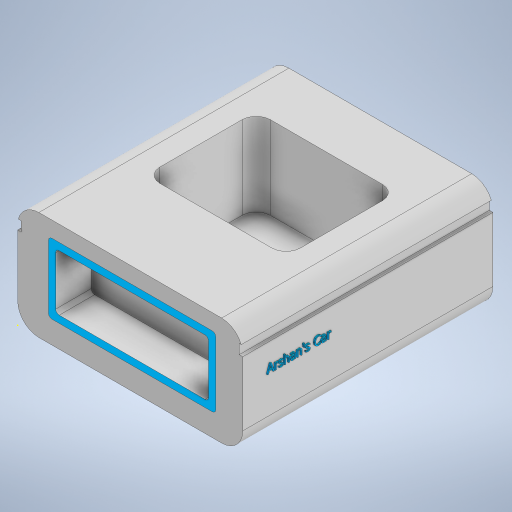
# Autodesk Inventor part: boxthing
Saved by Autodesk Inventor 2023 (Build 270158000, 158)
## iProperties
Created: 2023-08-29
Part Number: boxthing
Material: Generic
Document SubType Name: Modeling
Designer: 1908174
Density: 1 g/cm^3
Appearance: Default
Author: 1908174
Autodesk Inventor part; units mm, degrees
note: some values were not read from the file. Chosen so that the rebuilt part matches the saved one: direction of "Emboss1".
ref_plane "YZ Plane" through (0, 0, 0) normal (1, 0, 0) x (0, 1, 0)
ref_plane "XZ Plane" through (0, 0, 0) normal (0, 1, 0) x (-1, 0, 0)
ref_plane "XY Plane" through (0, 0, 0) normal (0, 0, 1) x (1, 0, 0)
sketch "Sketch2" plane through (0, 0, 0) normal (0, 1, 0) x (-1, 0, 0)
  line L0 (0, -89.780498) -> (-81.1276, -89.780498)
  line L1 (-81.1276, -89.780498) -> (-81.1276, 0.338702)
  line L2 (-81.1276, 0.338702) -> (0, 0.338702)
  line L3 (0, 0.338702) -> (0, -89.780498)
  point P0 (0, 0)
  dimension "d0" = 81.1276
  dimension "d1" = 90.1192
  constraints: 8 end point, 2 parallel, 1 horizontal, 1 perpendicular
  measures "d0" distance of L1.end L2.end
  measures "d1" distance of L0.end L1.end
extrude "Extrusion1" add sketch "Sketch2" along normal blind 39.0144
sketch "Sketch3" plane through (0, 39.0144, 0) normal (0, 1, 0) x (1, 0, 0)
  line L0 (15.2654, 70.349498) -> (65.8368, 70.349498)
  line L1 (65.8368, 70.349498) -> (65.8368, 30.573098)
  line L2 (65.8368, 30.573098) -> (15.2654, 30.573098)
  line L3 (15.2654, 30.573098) -> (15.2654, 70.349498)
  line L4 (0, -0.338702) -> (81.1276, -0.338702)
  line L5 (81.1276, -0.338702) -> (81.1276, 89.780498)
  point P0 (0, 0)
  dimension "d4" = 50.5714
  dimension "d5" = 39.7764
  dimension "d6" = 30.9118
  dimension "d7" = 15.2908
  constraints: 8 end point, 2 parallel, 1 horizontal, 1 perpendicular
  measures "d4" distance of L1.end L2.end
  measures "d5" distance of L0.end L1.end
  measures "d6" distance between parallel lines of L4 L2
  measures "d7" distance between parallel lines of L5 L1
extrude "Extrusion2" cut sketch "Sketch3" against normal blind 29.8704
sketch "Sketch4" plane through (0, 0, 0.338702) normal (0, 0, 1) x (1, 0, 0)
  line L0 (13.6906, 30.7594) -> (68.7832, 30.7594)
  line L1 (68.7832, 30.7594) -> (68.7832, 10.6426)
  line L2 (68.7832, 10.6426) -> (13.6906, 10.6426)
  line L3 (13.6906, 10.6426) -> (13.6906, 30.7594)
  line L4 (0, 0) -> (81.1276, 0) projected
  line L5 (0, 0) -> (0, 39.0144) projected
  dimension "d10" = 55.0926
  dimension "d11" = 20.1168
  dimension "d12" = 10.6426
  dimension "d13" = 13.6906
  constraints: 8 end point, 2 parallel, 1 horizontal, 1 perpendicular
  measures "d10" distance of L1.end L2.end
  measures "d11" distance of L0.end L1.end
  measures "d12" distance between parallel lines of L4 L2
  measures "d13" distance between parallel lines of L5 L3
extrude "Extrusion3" cut sketch "Sketch4" against normal blind 12.8016
sketch "Sketch5" plane through (81.1276, 0, -89.780498) normal (0, 0, -1) x (-1, 0, 0)
  line L0 (13.6906, 30.7594) -> (68.7832, 30.7594)
  line L1 (68.7832, 30.7594) -> (68.7832, 10.6426)
  line L2 (68.7832, 10.6426) -> (13.6906, 10.6426)
  line L3 (13.6906, 10.6426) -> (13.6906, 30.7594)
  line L4 (0, 0) -> (81.1276, 0)
  line L5 (0, 0) -> (0, 39.0144)
  dimension "d16" = 55.0926
  dimension "d17" = 20.1168
  dimension "d18" = 10.6426
  dimension "d19" = 13.6906
  constraints: 12 end point, 2 parallel, 1 horizontal, 1 perpendicular
  measures "d16" distance of L1.end L2.end
  measures "d17" distance of L0.end L1.end
  measures "d18" distance between parallel lines of L4 L2
  measures "d19" distance between parallel lines of L5 L3
extrude "Extrusion4" cut sketch "Sketch5" against normal blind 12.8016
fillet "Fillet3" radius 7.62 4 edges at (81.1276, 39.0144, -44.7209) (81.1276, 0, -44.7209) (0, 39.0144, -44.7209) (0, 0, -44.7209)
fillet "Fillet6" radius 5.08 8 edges at (15.2654, 24.0792, -30.5731) (65.8368, 24.0792, -70.3495) (15.2654, 24.0792, -70.3495) (65.8368, 24.0792, -30.5731) (67.437, 10.6426, -83.3797) (12.3444, 30.7594, -83.3797) (12.3444, 10.6426, -83.3797) (67.437, 30.7594, -83.3797)
sketch "Sketch6" plane through (7.62, 0, 0.338702) normal (0, 0, 1) x (1, 0, 0)
  line L0 (4.7244, 33.3248) -> (62.5094, 33.3248)
  line L1 (63.7794, 32.0548) -> (63.7794, 9.3472)
  line L2 (62.5094, 8.0772) -> (4.7244, 8.0772)
  line L3 (3.4544, 9.3472) -> (3.4544, 32.0548)
  line L4 (61.1632, 30.7594) -> (61.1632, 10.6426) projected
  line L5 (6.0706, 10.6426) -> (6.0706, 30.7594) projected
  line L6 (61.1632, 10.6426) -> (6.0706, 10.6426) projected
  line L7 (6.0706, 30.7594) -> (61.1632, 30.7594) projected
  arc A0 (3.4544, 9.3472) -> (4.7244, 8.0772) centre (4.7244, 9.3472) ccw
  arc A1 (4.7244, 33.3248) -> (3.4544, 32.0548) centre (4.7244, 32.0548) ccw
  arc A2 (63.7794, 32.0548) -> (62.5094, 33.3248) centre (62.5094, 32.0548) ccw
  arc A3 (62.5094, 8.0772) -> (63.7794, 9.3472) centre (62.5094, 9.3472) ccw
  point P0 (-7.62, 0)
  point P1 (3.4544, 33.3248)
  point P2 (63.7794, 8.0772)
  point P3 (63.7794, 33.3248)
  point P4 (3.4544, 8.0772)
  point P5 (61.1632, 25.6794)
  point P6 (61.1632, 15.7226)
  point P7 (6.0706, 15.7226)
  point P8 (6.0706, 25.6794)
  point P9 (56.0832, 10.6426)
  point P10 (11.1506, 10.6426)
  point P11 (11.1506, 30.7594)
  point P12 (56.0832, 30.7594)
  dimension "d28" = 2.6162
  dimension "d29" = 2.6162
  dimension "d30" = 2.5654
  dimension "d31" = 2.5654
  dimension "d34" = 1.27
  constraints: 8 end point, 8 point on circle, 8 point on line, 8 tangent, 4 centre point, 3 equal radius, 2 parallel, 1 horizontal, 1 perpendicular
  measures "d28" distance between parallel lines of L1 L4
  measures "d29" distance between parallel lines of L3 L5
  measures "d30" distance between parallel lines of L2 L6
  measures "d31" distance between parallel lines of L7 L0
  measures "d34" radius of A0
extrude "Extrusion5" cut sketch "Sketch6" against normal blind 0.000025 contours L0 A2 L1 A3 L2 A0 L3 A1 | L4 L6 L5 L7
fillet "Fillet7" radius 1.27 4 edges at (68.7832, 10.6426, -6.0621) (68.7832, 30.7594, -6.0621) (13.6906, 10.6426, -6.0621) (13.6906, 30.7594, -6.0621)
sketch "Sketch8" plane through (7.62, 0, 0.338702) normal (0, 0, 1) x (1, 0, 0)
  point P0 (-7.62, 0)
sketch "Sketch9" plane through (81.1276, 7.62, -89.780498) normal (1, 0, 0) x (0, 0, -1)
  line L0 (0, 18.0594) -> (0, 23.1394)
  line L1 (-90.617452, 26.634518) -> (0, 26.634518)
  line L2 (0, 26.634518) -> (0, 23.1394)
  line L3 (0, 23.1394) -> (-90.617452, 23.1394)
  line L4 (-90.617452, 23.1394) -> (-90.617452, 26.634518)
  point P0 (0, 23.1394)
  constraints: 10 end point, 2 parallel, 1 horizontal, 1 perpendicular
extrude "Extrusion6" [suppressed]
sketch "Sketch12" plane through (81.1276, 7.62, 0.338702) normal (1, 0, 0) x (0, 0, -1)
  line L0 (8.418749, 16.682779) -> (31.481291, 16.682779) construction
  line L1 (31.481291, 16.682779) -> (31.481291, 13.434708) construction
  line L2 (31.481291, 13.434708) -> (8.418749, 13.434708) construction
  line L3 (8.418749, 13.434708) -> (8.418749, 16.682779) construction
  line L4 (8.398989, 13.498928) -> (9.426516, 16.546928)
  line L5 (9.426516, 16.546928) -> (9.925459, 16.546928)
  line L6 (9.925459, 16.546928) -> (10.952986, 13.498928)
  line L7 (10.952986, 13.498928) -> (10.525673, 13.498928)
  line L8 (10.525673, 13.498928) -> (10.249031, 14.351084)
  line L9 (10.249031, 14.351084) -> (9.085654, 14.351084)
  line L10 (9.085654, 14.351084) -> (8.809012, 13.498928)
  line L11 (8.809012, 13.498928) -> (8.398989, 13.498928)
  line L12 (10.137881, 14.696886) -> (9.666108, 16.131966)
  line L13 (9.666108, 16.131966) -> (9.196805, 14.696886)
  line L14 (9.196805, 14.696886) -> (10.137881, 14.696886)
  line L15 (12.425116, 15.373671) -> (12.405356, 15.373671)
  spline S0 degree 2 poles (12.405356, 15.373671) (12.360895, 15.386021) (12.264565, 15.390961) (12.197874, 15.390961) knots 0 0 0 1 2 2 2
  spline S1 degree 2 poles (12.197874, 15.390961) (12.042263, 15.390961) (11.735981, 15.25511) (11.59766, 15.121729) knots 0 0 0 1 2 2 2
  line L16 (11.59766, 15.121729) -> (11.59766, 13.498928)
  line L17 (11.59766, 13.498928) -> (11.212338, 13.498928)
  line L18 (11.212338, 13.498928) -> (11.212338, 15.786163)
  line L19 (11.212338, 15.786163) -> (11.59766, 15.786163)
  line L20 (11.59766, 15.786163) -> (11.59766, 15.445301)
  spline S2 degree 2 poles (11.59766, 15.445301) (11.807612, 15.633022) (12.121304, 15.786163) (12.269505, 15.786163) knots 0 0 0 1 2 2 2
  spline S3 degree 2 poles (12.269505, 15.786163) (12.328785, 15.786163) (12.388065, 15.781223) (12.425116, 15.773813) knots 0 0 0 1 2 2 2
  line L21 (12.425116, 15.773813) -> (12.425116, 15.373671)
  spline S4 degree 2 poles (13.341492, 13.444588) (13.11178, 13.444588) (12.714108, 13.568089) (12.583197, 13.637249) knots 0 0 0 1 2 2 2
  line L22 (12.583197, 13.637249) -> (12.583197, 14.069502)
  line L23 (12.583197, 14.069502) -> (12.602957, 14.069502)
  spline S5 degree 2 poles (12.602957, 14.069502) (12.652357, 14.029982) (12.785738, 13.936121) (12.896889, 13.884251) knots 0 0 0 1 2 2 2
  spline S6 degree 2 poles (12.896889, 13.884251) (12.993219, 13.83732) (13.230341, 13.76816) (13.356312, 13.76816) knots 0 0 0 1 2 2 2
  spline S7 degree 2 poles (13.356312, 13.76816) (13.447702, 13.76816) (13.657654, 13.81015) (13.707054, 13.84473) knots 0 0 0 1 2 2 2
  spline S8 degree 2 poles (13.707054, 13.84473) (13.778685, 13.891661) (13.842905, 13.997871) (13.842905, 14.106552) knots 0 0 0 1 2 2 2
  spline S9 degree 2 poles (13.842905, 14.106552) (13.842905, 14.242403) (13.694704, 14.383194) (13.504513, 14.430124) knots 0 0 0 1 2 2 2
  spline S10 degree 2 poles (13.504513, 14.430124) (13.430412, 14.447414) (13.193291, 14.496815) (13.09202, 14.523985) knots 0 0 0 1 2 2 2
  spline S11 degree 2 poles (13.09202, 14.523985) (12.830198, 14.600555) (12.593077, 14.916718) (12.593077, 15.141489) knots 0 0 0 1 2 2 2
  spline S12 degree 2 poles (12.593077, 15.141489) (12.593077, 15.452711) (13.05991, 15.840504) (13.445232, 15.840504) knots 0 0 0 1 2 2 2
  spline S13 degree 2 poles (13.445232, 15.840504) (13.635424, 15.840504) (14.020746, 15.746643) (14.151657, 15.675013) knots 0 0 0 1 2 2 2
  line L24 (14.151657, 15.675013) -> (14.151657, 15.26252)
  line L25 (14.151657, 15.26252) -> (14.131897, 15.26252)
  spline S14 degree 2 poles (14.131897, 15.26252) (13.983696, 15.381081) (13.623074, 15.516931) (13.437822, 15.516931) knots 0 0 0 1 2 2 2
  spline S15 degree 2 poles (13.437822, 15.516931) (13.247631, 15.516931) (12.985809, 15.35638) (12.985809, 15.195829) knots 0 0 0 1 2 2 2
  spline S16 degree 2 poles (12.985809, 15.195829) (12.985809, 15.050098) (13.14142, 14.909307) (13.314322, 14.864847) knots 0 0 0 1 2 2 2
  spline S17 degree 2 poles (13.314322, 14.864847) (13.398302, 14.842617) (13.610724, 14.798157) (13.726814, 14.770987) knots 0 0 0 1 2 2 2
  spline S18 degree 2 poles (13.726814, 14.770987) (13.978756, 14.706766) (14.235638, 14.412834) (14.235638, 14.158423) knots 0 0 0 1 2 2 2
  spline S19 degree 2 poles (14.235638, 14.158423) (14.235638, 14.010222) (14.119547, 13.7484) (14.005926, 13.652069) knots 0 0 0 1 2 2 2
  spline S20 degree 2 poles (14.005926, 13.652069) (13.884895, 13.550799) (13.576143, 13.444588) (13.341492, 13.444588) knots 0 0 0 1 2 2 2
  line L26 (16.389492, 13.498928) -> (16.004169, 13.498928)
  line L27 (16.004169, 13.498928) -> (16.004169, 14.803097)
  spline S21 degree 2 poles (16.004169, 14.803097) (16.004169, 14.961178) (15.974529, 15.23288) (15.930069, 15.31439) knots 0 0 0 1 2 2 2
  spline S22 degree 2 poles (15.930069, 15.31439) (15.883138, 15.400841) (15.715177, 15.484821) (15.571916, 15.484821) knots 0 0 0 1 2 2 2
  spline S23 degree 2 poles (15.571916, 15.484821) (15.428655, 15.484821) (15.124843, 15.33168) (14.979113, 15.208179) knots 0 0 0 1 2 2 2
  line L28 (14.979113, 15.208179) -> (14.979113, 13.498928)
  line L29 (14.979113, 13.498928) -> (14.59379, 13.498928)
  line L30 (14.59379, 13.498928) -> (14.59379, 16.682779)
  line L31 (14.59379, 16.682779) -> (14.979113, 16.682779)
  line L32 (14.979113, 16.682779) -> (14.979113, 15.531752)
  spline S24 degree 2 poles (14.979113, 15.531752) (15.152014, 15.687363) (15.485466, 15.850384) (15.673187, 15.850384) knots 0 0 0 1 2 2 2
  spline S25 degree 2 poles (15.673187, 15.850384) (16.009109, 15.850384) (16.389492, 15.405781) (16.389492, 14.983408) knots 0 0 0 1 2 2 2
  line L33 (16.389492, 14.983408) -> (16.389492, 13.498928)
  spline S26 degree 2 poles (18.204954, 13.74099) (18.158023, 13.70641) (17.999942, 13.582909) (17.925842, 13.545859) knots 0 0 0 1 2 2 2
  spline S27 degree 2 poles (17.925842, 13.545859) (17.824571, 13.491518) (17.63438, 13.434708) (17.461479, 13.434708) knots 0 0 0 1 2 2 2
  spline S28 degree 2 poles (17.461479, 13.434708) (17.320688, 13.434708) (17.066276, 13.540918) (16.969946, 13.637249) knots 0 0 0 1 2 2 2
  spline S29 degree 2 poles (16.969946, 13.637249) (16.878555, 13.73111) (16.767404, 14.007752) (16.767404, 14.160893) knots 0 0 0 1 2 2 2
  spline S30 degree 2 poles (16.767404, 14.160893) (16.767404, 14.398014) (16.967476, 14.733936) (17.184837, 14.830267) knots 0 0 0 1 2 2 2
  spline S31 degree 2 poles (17.184837, 14.830267) (17.377498, 14.919188) (17.901142, 14.985878) (18.204954, 15.003168) knots 0 0 0 1 2 2 2
  line L34 (18.204954, 15.003168) -> (18.204954, 15.077269)
  spline S32 degree 2 poles (18.204954, 15.077269) (18.204954, 15.210649) (18.123443, 15.376141) (18.049343, 15.423071) knots 0 0 0 1 2 2 2
  spline S33 degree 2 poles (18.049343, 15.423071) (17.975242, 15.470001) (17.762821, 15.499641) (17.6492, 15.499641) knots 0 0 0 1 2 2 2
  spline S34 degree 2 poles (17.6492, 15.499641) (17.515819, 15.499641) (17.155197, 15.420601) (16.974886, 15.34403) knots 0 0 0 1 2 2 2
  line L35 (16.974886, 15.34403) -> (16.952655, 15.34403)
  line L36 (16.952655, 15.34403) -> (16.952655, 15.736763)
  spline S35 degree 2 poles (16.952655, 15.736763) (17.058866, 15.766403) (17.456539, 15.840504) (17.65167, 15.840504) knots 0 0 0 1 2 2 2
  spline S36 degree 2 poles (17.65167, 15.840504) (17.888792, 15.840504) (18.212364, 15.766403) (18.340805, 15.670072) knots 0 0 0 1 2 2 2
  spline S37 degree 2 poles (18.340805, 15.670072) (18.466775, 15.576212) (18.590276, 15.27734) (18.590276, 15.062448) knots 0 0 0 1 2 2 2
  line L37 (18.590276, 15.062448) -> (18.590276, 13.498928)
  line L38 (18.590276, 13.498928) -> (18.204954, 13.498928)
  line L39 (18.204954, 13.498928) -> (18.204954, 13.74099)
  line L40 (18.204954, 14.062092) -> (18.204954, 14.696886)
  spline S38 degree 2 poles (18.204954, 14.696886) (18.066633, 14.684536) (17.6492, 14.642546) (17.518289, 14.603025) knots 0 0 0 1 2 2 2
  spline S39 degree 2 poles (17.518289, 14.603025) (17.365148, 14.556095) (17.165077, 14.360964) (17.165077, 14.188063) knots 0 0 0 1 2 2 2
  spline S40 degree 2 poles (17.165077, 14.188063) (17.165077, 13.990461) (17.387378, 13.79039) (17.5998, 13.79039) knots 0 0 0 1 2 2 2
  spline S41 degree 2 poles (17.5998, 13.79039) (17.780111, 13.79039) (18.076513, 13.946001) (18.204954, 14.062092) knots 0 0 0 1 2 2 2
  line L41 (20.926912, 13.498928) -> (20.541589, 13.498928)
  line L42 (20.541589, 13.498928) -> (20.541589, 14.803097)
  spline S42 degree 2 poles (20.541589, 14.803097) (20.541589, 14.961178) (20.511949, 15.23288) (20.467489, 15.31439) knots 0 0 0 1 2 2 2
  spline S43 degree 2 poles (20.467489, 15.31439) (20.420558, 15.400841) (20.252597, 15.484821) (20.109336, 15.484821) knots 0 0 0 1 2 2 2
  spline S44 degree 2 poles (20.109336, 15.484821) (19.966075, 15.484821) (19.662263, 15.33168) (19.516532, 15.208179) knots 0 0 0 1 2 2 2
  line L43 (19.516532, 15.208179) -> (19.516532, 13.498928)
  line L44 (19.516532, 13.498928) -> (19.13121, 13.498928)
  line L45 (19.13121, 13.498928) -> (19.13121, 15.786163)
  line L46 (19.13121, 15.786163) -> (19.516532, 15.786163)
  line L47 (19.516532, 15.786163) -> (19.516532, 15.531752)
  spline S45 degree 2 poles (19.516532, 15.531752) (19.689433, 15.687363) (20.022886, 15.850384) (20.210607, 15.850384) knots 0 0 0 1 2 2 2
  spline S46 degree 2 poles (20.210607, 15.850384) (20.546529, 15.850384) (20.926912, 15.405781) (20.926912, 14.983408) knots 0 0 0 1 2 2 2
  line L48 (20.926912, 14.983408) -> (20.926912, 13.498928)
  line L49 (21.858108, 16.682779) -> (21.769187, 15.497171)
  line L50 (21.769187, 15.497171) -> (21.492545, 15.497171)
  line L51 (21.492545, 15.497171) -> (21.403625, 16.682779)
  line L52 (21.403625, 16.682779) -> (21.858108, 16.682779)
  spline S47 degree 2 poles (22.969615, 13.444588) (22.739904, 13.444588) (22.342231, 13.568089) (22.21132, 13.637249) knots 0 0 0 1 2 2 2
  line L53 (22.21132, 13.637249) -> (22.21132, 14.069502)
  line L54 (22.21132, 14.069502) -> (22.23108, 14.069502)
  spline S48 degree 2 poles (22.23108, 14.069502) (22.280481, 14.029982) (22.413861, 13.936121) (22.525012, 13.884251) knots 0 0 0 1 2 2 2
  spline S49 degree 2 poles (22.525012, 13.884251) (22.621343, 13.83732) (22.858464, 13.76816) (22.984435, 13.76816) knots 0 0 0 1 2 2 2
  spline S50 degree 2 poles (22.984435, 13.76816) (23.075826, 13.76816) (23.285777, 13.81015) (23.335177, 13.84473) knots 0 0 0 1 2 2 2
  spline S51 degree 2 poles (23.335177, 13.84473) (23.406808, 13.891661) (23.471028, 13.997871) (23.471028, 14.106552) knots 0 0 0 1 2 2 2
  spline S52 degree 2 poles (23.471028, 14.106552) (23.471028, 14.242403) (23.322827, 14.383194) (23.132636, 14.430124) knots 0 0 0 1 2 2 2
  spline S53 degree 2 poles (23.132636, 14.430124) (23.058536, 14.447414) (22.821414, 14.496815) (22.720143, 14.523985) knots 0 0 0 1 2 2 2
  spline S54 degree 2 poles (22.720143, 14.523985) (22.458322, 14.600555) (22.2212, 14.916718) (22.2212, 15.141489) knots 0 0 0 1 2 2 2
  spline S55 degree 2 poles (22.2212, 15.141489) (22.2212, 15.452711) (22.688033, 15.840504) (23.073356, 15.840504) knots 0 0 0 1 2 2 2
  spline S56 degree 2 poles (23.073356, 15.840504) (23.263547, 15.840504) (23.64887, 15.746643) (23.77978, 15.675013) knots 0 0 0 1 2 2 2
  line L55 (23.77978, 15.675013) -> (23.77978, 15.26252)
  line L56 (23.77978, 15.26252) -> (23.76002, 15.26252)
  spline S57 degree 2 poles (23.76002, 15.26252) (23.611819, 15.381081) (23.251197, 15.516931) (23.065946, 15.516931) knots 0 0 0 1 2 2 2
  spline S58 degree 2 poles (23.065946, 15.516931) (22.875754, 15.516931) (22.613933, 15.35638) (22.613933, 15.195829) knots 0 0 0 1 2 2 2
  spline S59 degree 2 poles (22.613933, 15.195829) (22.613933, 15.050098) (22.769544, 14.909307) (22.942445, 14.864847) knots 0 0 0 1 2 2 2
  spline S60 degree 2 poles (22.942445, 14.864847) (23.026425, 14.842617) (23.238847, 14.798157) (23.354938, 14.770987) knots 0 0 0 1 2 2 2
  spline S61 degree 2 poles (23.354938, 14.770987) (23.606879, 14.706766) (23.863761, 14.412834) (23.863761, 14.158423) knots 0 0 0 1 2 2 2
  spline S62 degree 2 poles (23.863761, 14.158423) (23.863761, 14.010222) (23.74767, 13.7484) (23.634049, 13.652069) knots 0 0 0 1 2 2 2
  spline S63 degree 2 poles (23.634049, 13.652069) (23.513019, 13.550799) (23.204267, 13.444588) (22.969615, 13.444588) knots 0 0 0 1 2 2 2
  spline S64 degree 2 poles (26.75121, 13.444588) (26.454808, 13.444588) (25.953395, 13.644659) (25.770613, 13.84473) knots 0 0 0 1 2 2 2
  spline S65 degree 2 poles (25.770613, 13.84473) (25.587832, 14.042332) (25.387761, 14.635136) (25.387761, 15.020458) knots 0 0 0 1 2 2 2
  spline S66 degree 2 poles (25.387761, 15.020458) (25.387761, 15.403311) (25.582892, 15.971414) (25.768143, 16.181366) knots 0 0 0 1 2 2 2
  spline S67 degree 2 poles (25.768143, 16.181366) (25.950925, 16.386377) (26.449868, 16.601269) (26.75862, 16.601269) knots 0 0 0 1 2 2 2
  spline S68 degree 2 poles (26.75862, 16.601269) (26.911761, 16.601269) (27.180993, 16.556808) (27.294613, 16.522228) knots 0 0 0 1 2 2 2
  spline S69 degree 2 poles (27.294613, 16.522228) (27.393414, 16.490118) (27.598425, 16.398727) (27.699696, 16.344387) knots 0 0 0 1 2 2 2
  line L57 (27.699696, 16.344387) -> (27.699696, 15.855324)
  line L58 (27.699696, 15.855324) -> (27.667586, 15.855324)
  spline S70 degree 2 poles (27.667586, 15.855324) (27.613246, 15.904724) (27.445284, 16.043045) (27.324254, 16.109735) knots 0 0 0 1 2 2 2
  spline S71 degree 2 poles (27.324254, 16.109735) (27.208163, 16.173956) (26.933991, 16.255466) (26.75615, 16.255466) knots 0 0 0 1 2 2 2
  spline S72 degree 2 poles (26.75615, 16.255466) (26.561019, 16.255466) (26.212746, 16.094915) (26.081836, 15.941774) knots 0 0 0 1 2 2 2
  spline S73 degree 2 poles (26.081836, 15.941774) (25.953395, 15.786163) (25.810134, 15.31439) (25.810134, 15.020458) knots 0 0 0 1 2 2 2
  spline S74 degree 2 poles (25.810134, 15.020458) (25.810134, 14.706766) (25.960805, 14.254753) (26.091716, 14.099142) knots 0 0 0 1 2 2 2
  spline S75 degree 2 poles (26.091716, 14.099142) (26.220156, 13.948471) (26.563489, 13.79533) (26.75615, 13.79533) knots 0 0 0 1 2 2 2
  spline S76 degree 2 poles (26.75615, 13.79533) (26.931521, 13.79533) (27.230393, 13.881781) (27.346484, 13.946001) knots 0 0 0 1 2 2 2
  spline S77 degree 2 poles (27.346484, 13.946001) (27.457635, 14.010222) (27.623126, 14.143602) (27.670056, 14.190533) knots 0 0 0 1 2 2 2
  line L59 (27.670056, 14.190533) -> (27.699696, 14.190533)
  line L60 (27.699696, 14.190533) -> (27.699696, 13.70641)
  spline S78 degree 2 poles (27.699696, 13.70641) (27.598425, 13.659479) (27.420584, 13.573029) (27.294613, 13.533508) knots 0 0 0 1 2 2 2
  spline S79 degree 2 poles (27.294613, 13.533508) (27.161233, 13.489048) (26.933991, 13.444588) (26.75121, 13.444588) knots 0 0 0 1 2 2 2
  spline S80 degree 2 poles (29.322497, 13.74099) (29.275567, 13.70641) (29.117485, 13.582909) (29.043385, 13.545859) knots 0 0 0 1 2 2 2
  spline S81 degree 2 poles (29.043385, 13.545859) (28.942114, 13.491518) (28.751923, 13.434708) (28.579022, 13.434708) knots 0 0 0 1 2 2 2
  spline S82 degree 2 poles (28.579022, 13.434708) (28.438231, 13.434708) (28.183819, 13.540918) (28.087489, 13.637249) knots 0 0 0 1 2 2 2
  spline S83 degree 2 poles (28.087489, 13.637249) (27.996098, 13.73111) (27.884947, 14.007752) (27.884947, 14.160893) knots 0 0 0 1 2 2 2
  spline S84 degree 2 poles (27.884947, 14.160893) (27.884947, 14.398014) (28.085019, 14.733936) (28.30238, 14.830267) knots 0 0 0 1 2 2 2
  spline S85 degree 2 poles (28.30238, 14.830267) (28.495041, 14.919188) (29.018685, 14.985878) (29.322497, 15.003168) knots 0 0 0 1 2 2 2
  line L61 (29.322497, 15.003168) -> (29.322497, 15.077269)
  spline S86 degree 2 poles (29.322497, 15.077269) (29.322497, 15.210649) (29.240986, 15.376141) (29.166886, 15.423071) knots 0 0 0 1 2 2 2
  spline S87 degree 2 poles (29.166886, 15.423071) (29.092785, 15.470001) (28.880364, 15.499641) (28.766743, 15.499641) knots 0 0 0 1 2 2 2
  spline S88 degree 2 poles (28.766743, 15.499641) (28.633362, 15.499641) (28.27274, 15.420601) (28.092429, 15.34403) knots 0 0 0 1 2 2 2
  line L62 (28.092429, 15.34403) -> (28.070199, 15.34403)
  line L63 (28.070199, 15.34403) -> (28.070199, 15.736763)
  spline S89 degree 2 poles (28.070199, 15.736763) (28.176409, 15.766403) (28.574082, 15.840504) (28.769213, 15.840504) knots 0 0 0 1 2 2 2
  spline S90 degree 2 poles (28.769213, 15.840504) (29.006335, 15.840504) (29.329907, 15.766403) (29.458348, 15.670072) knots 0 0 0 1 2 2 2
  spline S91 degree 2 poles (29.458348, 15.670072) (29.584319, 15.576212) (29.707819, 15.27734) (29.707819, 15.062448) knots 0 0 0 1 2 2 2
  line L64 (29.707819, 15.062448) -> (29.707819, 13.498928)
  line L65 (29.707819, 13.498928) -> (29.322497, 13.498928)
  line L66 (29.322497, 13.498928) -> (29.322497, 13.74099)
  line L67 (29.322497, 14.062092) -> (29.322497, 14.696886)
  spline S92 degree 2 poles (29.322497, 14.696886) (29.184176, 14.684536) (28.766743, 14.642546) (28.635832, 14.603025) knots 0 0 0 1 2 2 2
  spline S93 degree 2 poles (28.635832, 14.603025) (28.482691, 14.556095) (28.28262, 14.360964) (28.28262, 14.188063) knots 0 0 0 1 2 2 2
  spline S94 degree 2 poles (28.28262, 14.188063) (28.28262, 13.990461) (28.504921, 13.79039) (28.717343, 13.79039) knots 0 0 0 1 2 2 2
  spline S95 degree 2 poles (28.717343, 13.79039) (28.897654, 13.79039) (29.194056, 13.946001) (29.322497, 14.062092) knots 0 0 0 1 2 2 2
  line L68 (31.461531, 15.373671) -> (31.441771, 15.373671)
  spline S96 degree 2 poles (31.441771, 15.373671) (31.39731, 15.386021) (31.30098, 15.390961) (31.234289, 15.390961) knots 0 0 0 1 2 2 2
  spline S97 degree 2 poles (31.234289, 15.390961) (31.078678, 15.390961) (30.772396, 15.25511) (30.634075, 15.121729) knots 0 0 0 1 2 2 2
  line L69 (30.634075, 15.121729) -> (30.634075, 13.498928)
  line L70 (30.634075, 13.498928) -> (30.248753, 13.498928)
  line L71 (30.248753, 13.498928) -> (30.248753, 15.786163)
  line L72 (30.248753, 15.786163) -> (30.634075, 15.786163)
  line L73 (30.634075, 15.786163) -> (30.634075, 15.445301)
  spline S98 degree 2 poles (30.634075, 15.445301) (30.844027, 15.633022) (31.157719, 15.786163) (31.30592, 15.786163) knots 0 0 0 1 2 2 2
  spline S99 degree 2 poles (31.30592, 15.786163) (31.3652, 15.786163) (31.424481, 15.781223) (31.461531, 15.773813) knots 0 0 0 1 2 2 2
  line L74 (31.461531, 15.773813) -> (31.461531, 15.373671)
  point P0 (0.338702, -7.62)
  constraints: 2 other
emboss "Emboss1" sketch "Sketch12" operation add depth 0.508 direction (-1, 0, 0)
sketch "Sketch14" plane through (0, 6.624198, 0.562583) normal (-1, 0, 0) x (0, 0, 1)
  line L0 (0, 18.0594) -> (0, 23.1394)
  line L1 (-90.617452, 26.634518) -> (0, 26.634518)
  line L2 (0, 26.634518) -> (0, 23.1394)
  line L3 (0, 23.1394) -> (-90.617452, 23.1394)
  line L4 (-90.617452, 23.1394) -> (-90.617452, 26.634518)
  point P0 (-89.780498, -7.62)
  constraints: 10 end point, 2 parallel, 1 horizontal, 1 perpendicular
extrude "Extrusion9" cut sketch "Sketch14" against normal blind 1.27
sketch "Sketch15" plane through (81.1276, 7.62, -89.780498) normal (1, 0, 0) x (0, 0, -1)
  line L0 (0, 18.0594) -> (0, 23.1394)
  line L1 (-90.617452, 26.634518) -> (0, 26.634518)
  line L2 (0, 26.634518) -> (0, 23.1394)
  line L3 (0, 23.1394) -> (-90.617452, 23.1394)
  line L4 (-90.617452, 23.1394) -> (-90.617452, 26.634518)
  point P0 (-89.780498, -7.62)
  constraints: 10 end point, 2 parallel, 1 horizontal, 1 perpendicular
extrude "Extrusion10" cut sketch "Sketch15" against normal blind 1.27
body "Solid1"
